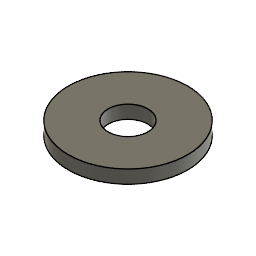
arruela_suporte_camadas_6mm_0-8mm (Autodesk Fusion 360 design; units mm, degrees)
Autodesk Fusion 360 part; units mm, degrees
sketch "Esboço1" plane through (0, 0, 0) normal (0, 1, 0) x (1, 0, 0)
  circle A0 centre (0, 0) radius 4.5
  circle A1 centre (0, 0) radius 1.5
  dimension "d1" = 9
  dimension "d2" = 3
  constraint coincident A0.centre A1.centre
  measures "d1" diameter of A0
  measures "d2" diameter of A1
extrude "Extrusão1" add sketch "Esboço1" along normal blind 1.5
extrude "Extrusão2" cut 1 faces at (3.4832, 1.5, 0.2236) along direction (0, -1, 0) blind 0.7
extrude "Extrusão3" add 1 faces at (3.4832, 0.8, 0.2236) along direction (0, 1, 0) blind 0.2
